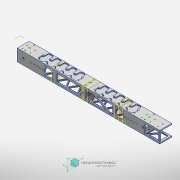
# Autodesk Inventor part: X-portal-front-plate
Saved by Autodesk Inventor 2016 (Build 200138000, 138)
## iProperties
Created: 2015-04-18
Part Number: X-portal-front-plate
Material: Aluminum 6061
Document SubType Name: Modeling
Designer: shu
Density: 2.7 g/cm^3
Appearance: Aluminum - Flat
Mass: 970.617 g
Surface Area: 2123.88 cm^2
Volume: 359.488 cm^3
Author: shu
Autodesk Inventor part; units mm, degrees
ref_plane "YZ Plane" through (0, 0, 0) normal (1, 0, 0) x (0, 1, 0)
ref_plane "XZ Plane" through (0, 0, 0) normal (0, 1, 0) x (-1, 0, 0)
ref_plane "XY Plane" through (0, 0, 0) normal (0, 0, 1) x (1, 0, 0)
sketch "Sketch1" plane through (0, 0, 0) normal (0, 0, 1) x (1, 0, 0)
  line L0 (0, 0) -> (800, 0)
  line L1 (800, 0) -> (800, -60)
  line L2 (800, -60) -> (0, -60)
  line L3 (0, -60) -> (0, 0)
  dimension "d0" = 800
  dimension "d1" = 60
  constraints: 8 end point, 2 parallel, 1 horizontal, 1 perpendicular
  measures "d0" distance of L1.end L2.end
  measures "d1" distance of L0.end L1.end
extrude "Extrusion1" add sketch "Sketch1" along normal blind 5
sketch "Sketch13" plane through (0, 0, 0) normal (0, 0, -1) x (-1, 0, 0)
  line L0 (0, -60) -> (-800, -60) projected
  line L1 (0, -60) -> (-800, -60)
  line L2 (-800, -60) -> (-800, -55)
  line L3 (-800, -55) -> (0, -55)
  line L4 (0, -55) -> (0, -60)
  point P0 (0, 0)
  dimension "d65" = 800
  dimension "d66" = 5
  constraints: 8 end point, 2 parallel, 1 horizontal, 1 perpendicular
  measures "d65" distance of L2.end L3.end
  measures "d66" distance of L1.end L2.end
extrude "Extrusion12" add sketch "Sketch13" along normal blind 55
sketch "Sketch14" plane through (0, 0, 5) normal (0, 0, 1) x (1, 0, 0)
  line L0 (60, 0) -> (60, -60) construction
  line L1 (0, -60) -> (800, -60) construction
  line L2 (0, -55) -> (0, 0) construction
  point P0 (60, -48)
  point P1 (60, -25)
  dimension "d71" = 60
  constraints: 3 point on line, 2 end point, 1 vertical
  measures "d71" distance from line of L2 point (60, -25)
hole "Hole1" at (60, -48, 5) at (60, -25, 5) direction (0, 0, -1) diameter 3.242 end through all thread size "M4x0.7" class "6H" standard "ISO Metric profile"
pattern_linear "Rectangular Pattern1" count 18 spacing 40 along (1, 0, 0) of "Hole1"
sketch "Sketch15" plane through (0, -55, -55) normal (0, 1, 0) x (1, 0, 0)
  line L0 (0, 0) -> (800, 0)
  line L1 (800, 0) -> (800, -5)
  line L2 (800, -5) -> (0, -5)
  line L3 (800, 0) -> (0, 0) projected
  line L4 (0, -5) -> (0, 0)
  line L5 (0, 0) -> (800, 0)
  line L6 (800, 0) -> (800, -5)
  constraints: 12 end point, 2 equal length, 2 perpendicular, 1 horizontal, 1 vertical
extrude "Extrusion13" add sketch "Sketch15" along normal up to surface (55 mm away)
sketch "Sketch20" plane through (0, 0, 5) normal (0, 0, 1) x (1, 0, 0)
  line L0 (0, 0) -> (21.0571, 0) construction
  line L1 (21.0571, 0) -> (21.0571, -30.3151) construction
  line L2 (21.0571, -30.3151) -> (0, -30.3151) construction
  line L3 (0, -30.3151) -> (0, 0) construction
  point P0 (75, -5)
  point P1 (375, -5)
  point P2 (675, -5)
  point P3 (75, -27.5)
  point P4 (375, -27.5)
  point P5 (675, -27.5)
  point P6 (75, -50)
  point P7 (375, -50)
  point P8 (675, -50)
  dimension "d123" = 300
  dimension "d126" = 22.5
  constraints: 8 end point, 2 horizontal, 2 parallel, 1 perpendicular, 1 vertical, 8 other
  measures "d123" distance of point (75, -5) point (375, -5)
  measures "d126" distance of point (75, -5) point (75, -27.5)
sketch "Sketch21" plane through (0, 0, 5) normal (0, 0, 1) x (1, 0, 0)
  point P0 (75, -50)
  point P1 (375, -27.5)
  point P2 (375, -50)
  point P3 (375, -5)
  point P4 (675, -5)
  point P5 (675, -27.5)
  point P6 (675, -50)
  point P7 (75, -5)
  point P8 (75, -27.5)
hole "Hole9" at (75, -50, 5) at (375, -27.5, 5) at (375, -50, 5) at (375, -5, 5) at (675, -5, 5) at (675, -27.5, 5) at (675, -50, 5) at (75, -5, 5) at (75, -27.5, 5) direction (0, 0, -1) diameter 5.5 depth 5
sketch "Sketch22" plane through (0, 0, -55) normal (0, 0, -1) x (-1, 0, 0)
  line L0 (0, 0) -> (-32.4648, 0) construction
  line L1 (-32.4648, 0) -> (-32.4648, -15.4297) construction
  line L2 (-32.4648, -15.4297) -> (0, -15.4297) construction
  line L3 (0, -15.4297) -> (0, 0) construction
  point P0 (-75, -5)
  point P1 (-375, -5)
  point P2 (-675, -5)
  point P3 (-75, -27.5)
  point P4 (-375, -27.5)
  point P5 (-675, -27.5)
  point P6 (-75, -50)
  point P7 (-375, -50)
  point P8 (-675, -50)
  dimension "d138" = 300
  dimension "d141" = 22.5
  constraints: 8 end point, 2 horizontal, 2 parallel, 1 perpendicular, 1 vertical, 8 other
  measures "d138" distance of point (-75, -5) point (-375, -5)
  measures "d141" distance of point (-75, -5) point (-75, -27.5)
hole "Hole11" at (75, -27.5, -55) at (75, -5, -55) at (75, -50, -55) at (375, -50, -55) at (375, -27.5, -55) at (375, -5, -55) at (675, -27.5, -55) at (675, -5, -55) at (675, -50, -55) direction (0, 0, 1) diameter 5 depth 5 tip angle 118
sketch "Sketch23" plane through (0, 0, 0) normal (0, 1, 0) x (1, 0, 0)
  point P0 (280, 52.5)
  point P1 (280, -2.5)
  point P2 (360, -2.5)
  point P3 (440, 52.5)
  point P4 (440, -2.5)
  point P5 (520, 52.5)
  point P6 (520, -2.5)
  point P7 (600, 52.5)
  point P8 (600, -2.5)
  point P9 (360, 52.5)
  point P10 (120, 52.5)
  point P11 (120, -2.5)
  point P12 (200, 52.5)
  point P13 (200, -2.5)
hole "Hole12" at (280, 0, -52.5) at (280, 0, 2.5) at (360, 0, 2.5) at (440, 0, -52.5) at (440, 0, 2.5) at (520, 0, -52.5) at (520, 0, 2.5) at (600, 0, -52.5) at (600, 0, 2.5) at (360, 0, -52.5) at (120, 0, -52.5) at (120, 0, 2.5) at (200, 0, -52.5) at (200, 0, 2.5) direction (0, -1, 0) diameter 2.459 depth 7 tip angle 120 thread size "M3x0.5" class "6H" standard "ISO Metric profile"
sketch "Sketch25" plane through (0, -55, 0) normal (0, 1, 0) x (1, 0, 0)
  point P0 (538, 44)
  point P1 (577, 44)
  point P2 (577, 6)
  point P3 (538, 6)
hole "Hole16" at (538, -55, -44) at (577, -55, -44) at (577, -55, -6) at (538, -55, -6) direction (0, -1, 0) diameter 5.5 depth 5
sketch "Sketch26" plane through (0, -55, 0) normal (0, 1, 0) x (1, 0, 0)
  point P0 (183, 44)
  point P1 (183, 6)
  point P2 (222, 6)
  point P3 (222, 44)
hole "Hole18" at (183, -55, -44) at (183, -55, -6) at (222, -55, -6) at (222, -55, -44) direction (0, -1, 0) diameter 5.5 depth 5
sketch "Sketch27" plane through (0, 0, -55) normal (0, 0, -1) x (-1, 0, 0)
  line L0 (-68, -55) -> (-82, -55) construction
  line L1 (-82, -55) -> (-82, 0) construction
  line L2 (-82, 0) -> (-68, 0) construction
  line L3 (-68, 0) -> (-68, -55) construction
  circle A0 centre (-75, -27.5) radius 2.5 construction
  line L4 (-68, -55) -> (-82, 0) construction
  line L5 (-82, -55) -> (-68, 0) construction
  line L6 (-368, -55) -> (-382, -55) construction
  line L7 (-382, -55) -> (-382, 0) construction
  line L8 (-382, 0) -> (-368, 0) construction
  line L9 (-368, 0) -> (-368, -55) construction
  line L10 (-368, -55) -> (-382, 0) construction
  line L11 (-382, -55) -> (-368, 0) construction
  line L12 (-668, -55) -> (-682, -55) construction
  line L13 (-682, -55) -> (-682, 0) construction
  line L14 (-682, 0) -> (-668, 0) construction
  line L15 (-668, 0) -> (-668, -55) construction
  line L16 (-668, -55) -> (-682, 0) construction
  line L17 (-682, -55) -> (-668, 0) construction
  line L18 (-95.0814, -41.5) -> (-115, -53) construction
  line L19 (-115, -53) -> (-134.9186, -41.5) construction
  line L20 (-134.9186, -41.5) -> (-134.9186, -18.5) construction
  line L21 (-134.9186, -18.5) -> (-115, -7) construction
  line L22 (-115, -7) -> (-95.0814, -18.5) construction
  line L23 (-95.0814, -18.5) -> (-95.0814, -41.5) construction
  line L24 (0, 0) -> (-800, 0) construction
  point P0 (-375, -27.5)
  point P1 (-675, -27.5)
  point P2 (-115, -30)
  dimension "d183" = 14
  dimension "d184" = 55
  dimension "d187" = 300
  dimension "d192" = 23
  dimension "d194" = 30
  dimension "d195" = 40
  constraints: 48 end point, 6 midpoint, 2 horizontal, 2 parallel, 1 collinear, 1 perpendicular, 34 other
  measures "d183" distance of L1.end L2.end
  measures "d184" distance of L0.end L1.end
  measures "d187" distance of L0.start L6.start
  measures "d192" distance of point (-115, -30) L21.end
  measures "d194" distance from line of L24 point (-115, -30)
  measures "d195" horizontal distance of point (-115, -30) A0.centre
sketch "Sketch38" plane through (0, -60, 5) normal (-1, 0, 0) x (0, 0, 1)
  line L0 (0, 0) -> (-60, 0)
  line L1 (-60, 0) -> (-60, 60)
  line L2 (-60, 60) -> (0, 60)
  line L3 (0, 60) -> (0, 0)
  point P0 (-5, 60)
  constraints: 8 end point, 2 parallel, 1 horizontal, 1 perpendicular
extrude "Extrusion19" cut sketch "Sketch38" against normal blind 45
ref_plane "Work Plane12" through (402.5, -55, 0) normal (1, 0, 0) x (0, 0, -1)
move faces "Move1" translate (-40, 0, 0) faces at (800, -38.3333, 3.3333)
sketch "Sketch28" plane through (0, 0, -55) normal (0, 0, -1) x (-1, 0, 0)
  line L0 (-126.0718, -8.2737) -> (-91.9282, -8.2737)
  line L1 (-88.4641, -14.2737) -> (-105.5359, -43.8429)
  line L2 (-112.4641, -43.8429) -> (-129.5359, -14.2737)
  line L3 (0, 0) -> (-800, 0) projected
  circle A0 centre (-75, -27.5) radius 2.5 projected
  line L4 (-158.5359, -43.8429) -> (-141.4641, -14.2737)
  line L5 (-134.5359, -14.2737) -> (-117.4641, -43.8429)
  line L6 (-120.9282, -49.8429) -> (-155.0718, -49.8429)
  circle A1 centre (-375, -27.5) radius 2.5 projected
  arc A2 (-134.5359, -14.2737) -> (-141.4641, -14.2737) centre (-138, -16.2737) ccw
  arc A3 (-158.5359, -43.8429) -> (-155.0718, -49.8429) centre (-155.0718, -45.8429) ccw
  arc A4 (-120.9282, -49.8429) -> (-117.4641, -43.8429) centre (-120.9282, -45.8429) ccw
  arc A5 (-126.0718, -8.2737) -> (-129.5359, -14.2737) centre (-126.0718, -12.2737) ccw
  arc A6 (-88.4641, -14.2737) -> (-91.9282, -8.2737) centre (-91.9282, -12.2737) ccw
  arc A7 (-112.4641, -43.8429) -> (-105.5359, -43.8429) centre (-109, -41.8429) ccw
  line L7 (-170.4641, -43.8429) -> (-187.5359, -14.2737)
  arc A8 (-184.0718, -8.2737) -> (-187.5359, -14.2737) centre (-184.0718, -12.2737) ccw
  arc A9 (-170.4641, -43.8429) -> (-163.5359, -43.8429) centre (-167, -41.8429) ccw
  arc A10 (-146.4641, -14.2737) -> (-149.9282, -8.2737) centre (-149.9282, -12.2737) ccw
  line L8 (-184.0718, -8.2737) -> (-149.9282, -8.2737)
  line L9 (-146.4641, -14.2737) -> (-163.5359, -43.8429)
  line L10 (-228.4641, -43.8429) -> (-245.5359, -14.2737)
  arc A11 (-242.0718, -8.2737) -> (-245.5359, -14.2737) centre (-242.0718, -12.2737) ccw
  arc A12 (-228.4641, -43.8429) -> (-221.5359, -43.8429) centre (-225, -41.8429) ccw
  arc A13 (-204.4641, -14.2737) -> (-207.9282, -8.2737) centre (-207.9282, -12.2737) ccw
  line L11 (-242.0718, -8.2737) -> (-207.9282, -8.2737)
  line L12 (-204.4641, -14.2737) -> (-221.5359, -43.8429)
  line L13 (-286.4641, -43.8429) -> (-303.5359, -14.2737)
  arc A14 (-300.0718, -8.2737) -> (-303.5359, -14.2737) centre (-300.0718, -12.2737) ccw
  arc A15 (-286.4641, -43.8429) -> (-279.5359, -43.8429) centre (-283, -41.8429) ccw
  arc A16 (-262.4641, -14.2737) -> (-265.9282, -8.2737) centre (-265.9282, -12.2737) ccw
  line L14 (-300.0718, -8.2737) -> (-265.9282, -8.2737)
  line L15 (-262.4641, -14.2737) -> (-279.5359, -43.8429)
  line L16 (-344.4641, -43.8429) -> (-361.5359, -14.2737)
  arc A17 (-358.0718, -8.2737) -> (-361.5359, -14.2737) centre (-358.0718, -12.2737) ccw
  arc A18 (-344.4641, -43.8429) -> (-337.5359, -43.8429) centre (-341, -41.8429) ccw
  arc A19 (-320.4641, -14.2737) -> (-323.9282, -8.2737) centre (-323.9282, -12.2737) ccw
  line L17 (-358.0718, -8.2737) -> (-323.9282, -8.2737)
  line L18 (-320.4641, -14.2737) -> (-337.5359, -43.8429)
  arc A20 (-192.5359, -14.2737) -> (-199.4641, -14.2737) centre (-196, -16.2737) ccw
  line L19 (-216.5359, -43.8429) -> (-199.4641, -14.2737)
  arc A21 (-216.5359, -43.8429) -> (-213.0718, -49.8429) centre (-213.0718, -45.8429) ccw
  line L20 (-178.9282, -49.8429) -> (-213.0718, -49.8429)
  line L21 (-192.5359, -14.2737) -> (-175.4641, -43.8429)
  arc A22 (-178.9282, -49.8429) -> (-175.4641, -43.8429) centre (-178.9282, -45.8429) ccw
  arc A23 (-250.5359, -14.2737) -> (-257.4641, -14.2737) centre (-254, -16.2737) ccw
  line L22 (-274.5359, -43.8429) -> (-257.4641, -14.2737)
  arc A24 (-274.5359, -43.8429) -> (-271.0718, -49.8429) centre (-271.0718, -45.8429) ccw
  line L23 (-236.9282, -49.8429) -> (-271.0718, -49.8429)
  line L24 (-250.5359, -14.2737) -> (-233.4641, -43.8429)
  arc A25 (-236.9282, -49.8429) -> (-233.4641, -43.8429) centre (-236.9282, -45.8429) ccw
  arc A26 (-308.5359, -14.2737) -> (-315.4641, -14.2737) centre (-312, -16.2737) ccw
  line L25 (-332.5359, -43.8429) -> (-315.4641, -14.2737)
  arc A27 (-332.5359, -43.8429) -> (-329.0718, -49.8429) centre (-329.0718, -45.8429) ccw
  line L26 (-294.9282, -49.8429) -> (-329.0718, -49.8429)
  line L27 (-308.5359, -14.2737) -> (-291.4641, -43.8429)
  arc A28 (-294.9282, -49.8429) -> (-291.4641, -43.8429) centre (-294.9282, -45.8429) ccw
  point P0 (-109, -22.1301)
  point P1 (-133, -8.2737)
  point P2 (-85, -8.2737)
  point P3 (-109, -49.8429)
  point P4 (-138, -35.9865)
  point P5 (-162, -49.8429)
  point P6 (-138, -8.2737)
  point P7 (-114, -49.8429)
  point P8 (-167, -22.1301)
  point P9 (-191, -8.2737)
  point P10 (-167, -49.8429)
  point P11 (-143, -8.2737)
  point P12 (-225, -22.1301)
  point P13 (-249, -8.2737)
  point P14 (-225, -49.8429)
  point P15 (-201, -8.2737)
  point P16 (-283, -22.1301)
  point P17 (-307, -8.2737)
  point P18 (-283, -49.8429)
  point P19 (-259, -8.2737)
  point P20 (-341, -22.1301)
  point P21 (-365, -8.2737)
  point P22 (-341, -49.8429)
  point P23 (-317, -8.2737)
  point P24 (-196, -8.2737)
  point P25 (-220, -49.8429)
  point P26 (-172, -49.8429)
  point P27 (-196, -35.9865)
  point P28 (-254, -8.2737)
  point P29 (-278, -49.8429)
  point P30 (-230, -49.8429)
  point P31 (-254, -35.9865)
  point P32 (-312, -8.2737)
  point P33 (-336, -49.8429)
  point P34 (-288, -49.8429)
  point P35 (-312, -35.9865)
  dimension "d196" = 10
  dimension "d197" = 48
  dimension "d209" = 48
  dimension "d210" = 41.5692
  dimension "d211" = 0
  dimension "d213" = 53
  dimension "d214" = 4
  dimension "d215" = 4
  dimension "d218" = 58
  dimension "d225" = 58
  constraints: 54 end point, 54 point on circle, 54 point on line, 27 centre point, 12 tangent, 4 equal radius, 2 horizontal, 2 parallel, 147 other
  measures "d196" horizontal distance of A0.centre point (-85, -8.274)
  measures "d197" distance of point (-133, -8.274) point (-85, -8.274)
  measures "d209" distance of point (-162, -49.843) point (-138, -8.274)
  measures "d210" distance from line of point (-109, -49.843) L0
  measures "d211" distance from line of L0 point (-138, -8.274)
  measures "d213" distance of point (-85, -8.274) point (-138, -8.274)
  measures "d214" radius of A2
  measures "d215" radius of A5
  measures "d218" distance of point (-109, -22.13) point (-167, -22.13)
  measures "d225" distance of point (-138, -8.274) point (-196, -8.274)
extrude "Extrusion14" cut sketch "Sketch28" against normal blind 5 contours L0 A6 L1 A7 L2 A5 | L4 A2 L5 A4 L6 A3 | L7 A8 L8 A10 L9 A9 | L10 A11 L11 A13 L12 A12 | L13 A14 L14 A16 L15 A15 | L16 A17 L17 A19 L18 A18 | L21 A22 L20 A21 L19 A20 | L24 A25 L23 A24 L22 A23 | L27 A28 L26 A27 L25 A26
pattern_linear "Rectangular Pattern2" count 2 spacing 300 along (1, 0, 0) of "Extrusion14"
sketch "Sketch30" plane through (0, -60, 5) normal (0, -1, 0) x (1, 0, 0)
  line L0 (202.0191, -9) -> (202.0191, -51) construction
  line L1 (510.684, -51) -> (518.5, -51)
  line L2 (522, -47.5) -> (522, -12.5) construction
  line L3 (518.5, -9) -> (450.0622, -9) construction
  circle A0 centre (538, -49) radius 2.75 projected
  circle A1 centre (222, -49) radius 2.75 projected
  line L4 (800, -60) -> (0, -60) projected
  line L5 (0, 0) -> (800, 0) projected
  line L6 (433, -9) -> (505.7461, -51) construction
  line L7 (505.7461, -51) -> (433, -51) construction
  line L8 (508.934, -50.5311) -> (448.3122, -15.5311)
  line L9 (518.5, -9) -> (450.0622, -9)
  line L10 (518.5, -51) -> (509.7461, -51)
  line L11 (522, -47.5) -> (522, -12.5)
  arc A2 (450.0622, -9) -> (448.3122, -15.5311) centre (450.0622, -12.5) ccw
  arc A3 (522, -12.5) -> (518.5, -9) centre (518.5, -12.5) ccw
  arc A4 (518.5, -51) -> (522, -47.5) centre (518.5, -47.5) ccw
  arc A5 (508.934, -50.5311) -> (510.684, -51) centre (510.684, -47.5) ccw
  line L12 (425.1449, -11.0698) -> (390.5, -11.0698)
  line L13 (387, -14.5698) -> (387, -47.5) construction
  line L14 (390.5, -51) -> (482.1818, -51) construction
  line L15 (499.2439, -51) -> (430.0828, -11.0698) construction
  line L16 (430.0828, -11.0698) -> (410.6711, -11.0698) construction
  line L17 (426.8949, -11.5387) -> (483.9318, -44.4689)
  line L18 (390.5, -51) -> (482.1818, -51)
  line L19 (390.5, -11.0698) -> (426.0828, -11.0698)
  line L20 (387, -14.5698) -> (387, -47.5)
  arc A6 (482.1818, -51) -> (483.9318, -44.4689) centre (482.1818, -47.5) ccw
  arc A7 (387, -47.5) -> (390.5, -51) centre (390.5, -47.5) ccw
  arc A8 (390.5, -11.0698) -> (387, -14.5698) centre (390.5, -14.5698) ccw
  arc A9 (426.8949, -11.5387) -> (425.1449, -11.0698) centre (425.1449, -14.5698) ccw
  point P0 (0, -5)
  dimension "d251" = 42
  dimension "d252" = 320
  dimension "d253" = 16
  dimension "d254" = 19.9809
  dimension "d255" = 9
  dimension "d256" = 9
  dimension "d260" = 2
  dimension "d265" = 150
  dimension "d355" = 2
  dimension "d356" = 3.5
  dimension "d357" = 150
  dimension "d358" = 3.5
  dimension "d359" = 3.5
  dimension "d360" = 0
  dimension "d361" = 135
  constraints: 38 end point, 16 point on circle, 16 tangent, 10 point on line, 8 centre point, 3 parallel, 3 perpendicular, 2 collinear, 1 vertical
  measures "d251" distance of L0.start L0.end
  measures "d252" distance of L2.start L0.end
  measures "d253" distance from line of A0.centre L2
  measures "d254" distance from line of L0 A1.centre
  measures "d255" distance between parallel lines of L4 L1
  measures "d256" distance between parallel lines of L5 L3
  measures "d260" distance between parallel lines of L6 L8
  measures "d265" angle of L5 L8
  measures "d355" distance between parallel lines of L15 L17
  measures "d356" distance from line of A8.centre L20
  measures "d357" angle of L17 L19
  measures "d358" distance from line of L17 A6.centre
  measures "d359" distance from line of L18 A6.centre
  measures "d360" distance between parallel lines of L1 L14
  measures "d361" distance between parallel lines of L2 L13
extrude "Extrusion15" cut sketch "Sketch30" against normal blind 5 contours A5 L8 A2 L9 A3 L11 A4 L1 | A9 L17 A6 L18 A7 L20 A8 L12
ref_plane "Work Plane1" through (375, -50, -55) normal (-1, 0, 0) x (0, 0, 1)
ref_plane "Work Plane3" through (538, -60, -44) normal (1, 0, 0) x (0, 0, -1)
ref_plane "Work Plane4" through (557.5, -60, -44) normal (1, 0, 0) x (0, 0, -1)
ref_plane "Work Plane2" through (577, -60, -44) normal (1, 0, 0) x (0, 0, -1)
sketch "Sketch32" plane through (0, -60, 5) normal (0, -1, 0) x (1, 0, 0)
  line L0 (800, -5) -> (0, -5) projected
  line L1 (682.8407, -49.0155) -> (682.8407, -13.5)
  line L2 (686.3407, -10) -> (749.4795, -10)
  line L3 (751.1954, -16.5505) -> (688.0566, -52.066)
  arc A0 (751.1954, -16.5505) -> (749.4795, -10) centre (749.4795, -13.5) ccw
  arc A1 (686.3407, -10) -> (682.8407, -13.5) centre (686.3407, -13.5) ccw
  arc A2 (682.8407, -49.0155) -> (688.0566, -52.066) centre (686.3407, -49.0155) ccw
  line L4 (686.3407, -52.5155) -> (752.8652, -52.5155) construction
  line L5 (752.8652, -49.3155) -> (752.8652, -26.987)
  line L6 (748.0964, -24.198) -> (708.4013, -46.5265)
  line L7 (749.6652, -52.5155) -> (709.9701, -52.5155)
  arc A3 (749.6652, -52.5155) -> (752.8652, -49.3155) centre (749.6652, -49.3155) ccw
  arc A4 (752.8652, -26.987) -> (748.0964, -24.198) centre (749.6652, -26.987) ccw
  arc A5 (708.4013, -46.5265) -> (709.9701, -52.5155) centre (709.9701, -49.3155) ccw
  point P0 (682.8407, -55)
  point P1 (682.8407, -10)
  point P2 (762.8407, -10)
  point P3 (752.8652, -21.5155)
  point P4 (697.7541, -52.5155)
  dimension "d293" = 45
  dimension "d294" = 80
  dimension "d295" = 3.5
  dimension "d320" = 31
  dimension "d321" = 3.2
  constraints: 14 end point, 13 point on circle, 13 point on line, 12 tangent, 6 centre point, 4 equal radius, 2 parallel, 2 vertical, 1 collinear, 1 horizontal, 1 perpendicular
  measures "d293" distance of point (682.841, -55) point (682.841, -10)
  measures "d294" distance of point (682.841, -10) point (762.841, -10)
  measures "d295" radius of A0
  measures "d320" distance of L4.end point (752.865, -21.516)
  measures "d321" radius of A3
extrude "Extrusion16" cut sketch "Sketch32" against normal blind 5
sketch "Sketch33" plane through (0, -60, 5) normal (0, -1, 0) x (1, 0, 0)
  point P0 (0, -5)
sketch "Sketch39" plane through (45, -60, -55) normal (0, -1, 0) x (1, 0, 0)
  line L0 (330, -12) -> (330, 72) projected
  line L1 (314.5, 9) -> (201.5, 9)
  line L2 (198, 12.5) -> (198, 45.4302)
  line L3 (201.5, 48.9302) -> (314.5, 48.9302)
  line L4 (318, 45.4302) -> (318, 12.5)
  arc A0 (314.5, 9) -> (318, 12.5) centre (314.5, 12.5) ccw
  arc A1 (318, 45.4302) -> (314.5, 48.9302) centre (314.5, 45.4302) ccw
  arc A2 (198, 12.5) -> (201.5, 9) centre (201.5, 12.5) ccw
  arc A3 (201.5, 48.9302) -> (198, 45.4302) centre (201.5, 45.4302) ccw
  line L5 (345.5, 48.9302) -> (380.1449, 48.9302) projected
  line L6 (437.1818, 9) -> (345.5, 9) projected
  point P0 (-45, 55)
  dimension "d322" = 3.5
  dimension "d325" = 120
  dimension "d326" = 12
  dimension "d362" = 0
  dimension "d363" = 0
  constraints: 8 end point, 8 point on circle, 8 tangent, 4 centre point, 3 equal radius, 2 parallel, 1 horizontal, 1 perpendicular
  measures "d322" radius of A0
  measures "d325" distance between parallel lines of L2 L4
  measures "d326" distance between parallel lines of L0 L4
  measures "d362" distance between parallel lines of L5 L3
  measures "d363" distance between parallel lines of L6 L1
extrude "Extrusion20" cut sketch "Sketch39" against normal blind 5
sketch "Sketch40" plane through (0, 0, 5) normal (0, 0, 1) x (1, 0, 0)
  line L0 (140, -43.5) -> (140, -29.5)
  line L1 (140, -29.5) -> (180, -43.5) construction
  line L2 (180, -29.5) -> (140, -43.5) construction
  line L3 (160, -54.9) -> (150, -54.9)
  line L4 (146.8119, -20.3226) -> (175, -54.9) construction
  line L5 (173.1881, -20.3226) -> (145, -54.9) construction
  circle A0 centre (140, -25) radius 1.621 projected
  circle A1 centre (140, -48) radius 1.621 projected
  line L6 (160, 6) -> (160, -68)
  line L7 (146.8119, -20.3226) -> (146.8119, -10.25)
  line L8 (153.8119, -3.25) -> (160, -3.25)
  line L9 (760, 0) -> (45, 0) projected
  line L10 (140, -29.5) -> (142.5619, -29.5)
  line L11 (146.5574, -25.6895) -> (146.8119, -20.3226)
  line L12 (145, -49.9) -> (145, -47.5)
  line L13 (141, -43.5) -> (140, -43.5)
  arc A2 (142.5619, -29.5) -> (146.5574, -25.6895) centre (142.5619, -25.5) ccw
  arc A3 (145, -47.5) -> (141, -43.5) centre (141, -47.5) ccw
  arc A4 (145, -49.9) -> (150, -54.9) centre (150, -49.9) ccw
  arc A5 (153.8119, -3.25) -> (146.8119, -10.25) centre (153.8119, -10.25) ccw
  line L14 (180, -43.5) -> (180, -29.5)
  line L15 (160, -54.9) -> (170, -54.9)
  line L16 (173.1881, -20.3226) -> (173.1881, -10.25)
  line L17 (166.1881, -3.25) -> (160, -3.25)
  line L18 (180, -29.5) -> (177.4381, -29.5)
  line L19 (173.4426, -25.6895) -> (173.1881, -20.3226)
  line L20 (175, -49.9) -> (175, -47.5)
  line L21 (179, -43.5) -> (180, -43.5)
  arc A6 (173.4426, -25.6895) -> (177.4381, -29.5) centre (177.4381, -25.5) ccw
  arc A7 (179, -43.5) -> (175, -47.5) centre (179, -47.5) ccw
  arc A8 (170, -54.9) -> (175, -49.9) centre (170, -49.9) ccw
  arc A9 (173.1881, -10.25) -> (166.1881, -3.25) centre (166.1881, -10.25) ccw
  line L22 (45, -60) -> (760, -60) projected
  point P0 (0, 0)
  point P1 (160, -36.5)
  point P2 (160, -36.5)
  dimension "d329" = 40
  dimension "d331" = 30
  dimension "d333" = 40
  dimension "d334" = 0
  dimension "d335" = 11.5
  dimension "d336" = 23
  dimension "d337" = 4
  dimension "d338" = 5
  dimension "d339" = 7
  dimension "d340" = 5.1
  dimension "d341" = 26.3761
  dimension "d342" = 6.5
  dimension "d343" = 40
  constraints: 42 end point, 16 point on circle, 12 symmetric about line, 8 centre point, 8 point on line, 8 tangent, 3 midpoint, 2 coincident, 2 parallel, 2 vertical, 1 equal radius, 1 horizontal, 4 other
  measures "d329" distance of L1.end L0.start
  measures "d331" distance of L4.end L5.end
  measures "d333" diameter of point (140, -25) L6
  measures "d334" distance from line of point (160, -36.5) L6
  measures "d335" vertical distance of point (160, -36.5) A0.centre
  measures "d336" distance of point (140, -25) point (140, -48)
  measures "d337" radius of A2
  measures "d338" radius of A4
  measures "d339" radius of A5
  measures "d340" distance between parallel lines of L22 L3
  measures "d341" distance between parallel lines of L7 L16
  measures "d342" diameter of L8.end L9
  measures "d343" distance between parallel lines of L14 L0
extrude "Extrusion21" cut sketch "Sketch40" against normal blind 4.2 contours L0 L10 A2 L11 L7 A5 L8 L6 L3 A4 L12 A3 L13 | L6 L17 A9 L16 L19 A6 L18 L14 L21 A7 L20 A8 L15
pattern_linear "Rectangular Pattern3" count 5 spacing 40 along (1, 0, 0) of "Extrusion21"
pattern_linear "Rectangular Pattern4" count 2 spacing 280 along (1, 0, 0) of "Extrusion21", "Rectangular Pattern3"
sketch "Sketch41" plane through (45, -60, -55) normal (0, -1, 0) x (1, 0, 0)
  point P0 (630, 30)
hole "Hole20" at (675, -60, -25) direction (0, 1, 0) diameter 5.5 depth 5 counterbore diameter 10 counterbore depth 3.7
pattern_linear "Rectangular Pattern6" count 3 spacing 300 along (-1, 0, 0) of "Hole20"
sketch "Sketch42" plane through (45, -60, -55) normal (0, -1, 0) x (1, 0, 0)
  line L0 (512.5, 72) -> (512.5, -12) projected
  circle A0 centre (493, 11) radius 2.75 projected
  circle A1 centre (493, 49) radius 2.75 projected
  circle A2 centre (512.5, 30) radius 20
  point P0 (-45, 55)
  dimension "d374" = 38
  dimension "d375" = 40
  dimension "d376" = 19
  constraints: 1 centre point, 1 midpoint
  measures "d374" distance of A0.centre A1.centre
  measures "d375" diameter of A2
  measures "d376" vertical distance of A1.centre A2.centre
extrude "Extrusion22" cut sketch "Sketch42" against normal blind 5 contours A2 L0 | L0 A2
ref_plane "Midplane between Y columns" through (380, -60, -6) normal (1, 0, 0) x (0, 0, -1)
ref_plane "Work Plane9" through (222, -60, -6) normal (1, 0, 0) x (0, 0, -1)
mirror "Mirror4" about plane through (380, -60, -6) normal (1, 0, 0) of "Extrusion22"
sketch "Sketch43" plane through (45, -60, -55) normal (0, -1, 0) x (1, 0, 0)
  line L0 (0, 60) -> (715, 60) projected
  circle A0 centre (532, 49) radius 2.75 projected
  point P0 (-45, 55)
  point P1 (542, 30)
  point P2 (557, 30)
  point P3 (572, 30)
  point P4 (587, 30)
  point P5 (602, 30)
  dimension "d382" = 30
  dimension "d383" = 10
  dimension "d387" = 15
  constraints: 1 horizontal, 4 other
  measures "d382" distance from line of L0 point (542, 30)
  measures "d383" horizontal distance of A0.centre point (542, 30)
  measures "d387" distance of point (542, 30) point (557, 30)
hole "Hole22" at (587, -60, -25) at (602, -60, -25) at (617, -60, -25) at (632, -60, -25) at (647, -60, -25) direction (0, 1, 0) diameter 5.2 end through all
mirror "Mirror5" about plane through (380, -60, -6) normal (1, 0, 0) of "Hole22"
sketch "Sketch44" plane through (0, 0, -55) normal (0, 0, -1) x (-1, 0, 0)
  line L0 (-745.9, -49.8429) -> (-689.1, -49.8429)
  line L1 (-685, -45.7429) -> (-685, -12.3737)
  line L2 (-689.1, -8.2737) -> (-745.9, -8.2737)
  line L3 (-750, -12.3737) -> (-750, -45.7429)
  line L4 (-750, -49.8429) -> (-685, -8.2737) construction
  line L5 (-685, -49.8429) -> (-750, -8.2737) construction
  line L6 (-658.0718, -8.2737) -> (-623.9282, -8.2737) projected
  line L7 (-594.9282, -49.8429) -> (-629.0718, -49.8429) projected
  line L8 (-760, -60) -> (-760, 0) projected
  circle A0 centre (-675, -27.5) radius 2.5 projected
  arc A1 (-745.9, -8.2737) -> (-750, -12.3737) centre (-745.9, -12.3737) ccw
  arc A2 (-750, -45.7429) -> (-745.9, -49.8429) centre (-745.9, -45.7429) ccw
  arc A3 (-689.1, -49.8429) -> (-685, -45.7429) centre (-689.1, -45.7429) ccw
  arc A4 (-685, -12.3737) -> (-689.1, -8.2737) centre (-689.1, -12.3737) ccw
  point P0 (0, 0)
  point P1 (-717.5, -29.0583)
  dimension "d399" = 0
  dimension "d400" = 0
  dimension "d401" = 10
  dimension "d402" = 10
  dimension "d403" = 4.1
  constraints: 12 end point, 8 point on circle, 8 point on line, 8 tangent, 4 centre point, 3 equal radius, 2 midpoint, 2 parallel, 1 horizontal, 1 perpendicular
  measures "d399" distance between parallel lines of L6 L2
  measures "d400" distance between parallel lines of L7 L0
  measures "d401" distance between parallel lines of L8 L3
  measures "d402" distance from line of A0.centre L1
  measures "d403" radius of A1
extrude "Extrusion23" cut sketch "Sketch44" against normal blind 5 contours A2 L3 A1 L2 A4 L1 A3 L0
sketch "Sketch45" plane through (45, 0, 0) normal (0, 1, 0) x (1, 0, 0)
  line L0 (0, 0) -> (715, 0) projected
  line L1 (0, 0) -> (0, -5) projected
  point P0 (-45, 0)
  point P1 (6, -2.5)
  point P2 (21, -2.5)
  point P3 (36, -2.5)
  point P4 (51, -2.5)
  point P5 (66, -2.5)
  point P6 (6, 52.5)
  point P7 (21, 52.5)
  point P8 (36, 52.5)
  point P9 (51, 52.5)
  point P10 (66, 52.5)
  dimension "d406" = 6
  dimension "d407" = 2.5
  dimension "d410" = 15
  dimension "d413" = 55
  constraints: 1 horizontal, 1 vertical, 9 other
  measures "d406" distance from line of L1 point (6, -2.5)
  measures "d407" distance from line of point (6, -2.5) L0
  measures "d410" distance of point (6, -2.5) point (21, -2.5)
  measures "d413" distance of point (6, -2.5) point (6, 52.5)
hole "Hole23" at (51, 0, -52.5) at (66, 0, -52.5) at (81, 0, -52.5) at (96, 0, -52.5) at (111, 0, -52.5) at (51, 0, 2.5) at (66, 0, 2.5) at (81, 0, 2.5) at (96, 0, 2.5) at (111, 0, 2.5) direction (0, -1, 0) diameter 2.459 depth 10 tip angle 118 thread size "M3x0.5" class "6H" standard "ISO Metric profile"
ref_plane "Midplane whole part" through (402.5, -55, 0) normal (1, 0, 0) x (0, 0, -1)
mirror "Mirror6" about plane through (402.5, -55, 0) normal (1, 0, 0) of "Hole23"
equation "\"d183\" = d181"
equation "\"d209\" = d197"
equation "\"d213\" = d197 + 0.5 * d196"
equation "\"d218\" = d197 + d196"
equation "\"d225\" = d218"
equation "\"d181\" = 14"
body "Solid1" dims "d251" = 42, "d252" = 320, "d253" = 16, "d254" = 19.98086 (derived), "d255" = 9, "d256" = 9 (derived), "d260" = 2, "d265" = 150 deg, "d355" = 2, "d356" = 3.5, "d357" = 150 deg, "d358" = 3.5, "d359" = 3.5 (derived), "d360" = 0, "d361" = 135
